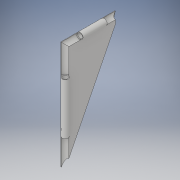
# Autodesk Inventor part: backPlate
Saved by Autodesk Inventor 2019 (Build 230136000, 136)
## iProperties
Created: 2018-07-23
Part Number: backPlate
Material: Generic
Document SubType Name: Modeling
Designer: Ge Shi
Density: 1 g/cm^3
Appearance: Default
Author: Ge Shi
Autodesk Inventor part; units mm, degrees
ref_plane "YZ Plane" through (0, 0, 0) normal (1, 0, 0) x (0, 1, 0)
ref_plane "XZ Plane" through (0, 0, 0) normal (0, 1, 0) x (-1, 0, 0)
ref_plane "XY Plane" through (0, 0, 0) normal (0, 0, 1) x (1, 0, 0)
sketch "Sketch1" plane through (0, 0, 0) normal (1, 0, 0) x (0, 1, 0)
  line L0 (-50, -25) -> (50, -25)
  line L1 (50, -25) -> (50, 25)
  line L2 (50, 25) -> (-50, 25)
  line L3 (-50, 25) -> (-50, -25)
  line L4 (-50, -25) -> (50, 25) construction
  line L5 (50, -25) -> (-50, 25) construction
  point P0 (0, 0)
  dimension "d0" = 50
  dimension "d1" = 100
  constraints: 12 end point, 2 midpoint, 2 parallel, 1 horizontal, 1 perpendicular
  measures "d0" distance of L0.end L1.end
  measures "d1" distance of L1.end L2.end
extrude "Extrusion1" add sketch "Sketch1" along normal blind 4
ref_plane "Work Plane1" through (0, 0, 25) normal (0, 1, 0) x (1, 0, 0)
ref_plane "Work Plane2" through (0, -50, 0) normal (0, 0, 1) x (1, 0, 0)
sketch "Sketch3" plane through (0, -50, 0) normal (0, 0, 1) x (1, 0, 0)
  circle A0 centre (4, 100) radius 2.25
  circle A1 centre (4, 0) radius 2.25
  circle A2 centre (4, 0) radius 2.75
  circle A3 centre (4, 100) radius 2.75
  line L0 (4, 0) -> (4, 100) projected
  circle A4 centre (4, 0) radius 3.5
  circle A5 centre (4, 100) radius 3.5
  point P0 (0, 50)
  dimension "d12" = 4.5
  dimension "d13" = 4.5
  dimension "d14" = 5.5
  dimension "d15" = 5.5
  dimension "d24" = 7
  dimension "d25" = 7
  constraints: 6 centre point, 4 coincident
  measures "d12" diameter of A0
  measures "d13" diameter of A1
  measures "d14" diameter of A2
  measures "d15" diameter of A3
  measures "d24" diameter of A4
  measures "d25" diameter of A5
sketch "Sketch2" plane through (0, 0, 25) normal (0, 1, 0) x (1, 0, 0)
  line L0 (4, 50) -> (4, 0) projected
  circle A0 centre (4, 0) radius 2.25
  circle A1 centre (4, 50) radius 2.25
  circle A2 centre (4, 0) radius 2.75
  circle A3 centre (4, 50) radius 2.75
  circle A4 centre (4, 0) radius 3.5
  circle A5 centre (4, 50) radius 3.5
  point P0 (0, 25)
  dimension "d4" = 4.5
  dimension "d5" = 4.5
  dimension "d6" = 5.5
  dimension "d7" = 5.5
  dimension "d20" = 7
  dimension "d21" = 7
  constraints: 6 centre point, 5 coincident
  measures "d4" diameter of A0
  measures "d5" diameter of A1
  measures "d6" diameter of A2
  measures "d7" diameter of A3
  measures "d20" diameter of A4
  measures "d21" diameter of A5
ref_plane "Work Plane4" through (0, -50, 25) normal (0, 0.4472136, 0.8944272) x (1, 0, 0)
extrude "Extrusion6" cut sketch "Sketch2" along normal mid plane 100 contours A0 | A1 | A2 | A3
extrude "Extrusion2" add sketch "Sketch2" along normal mid plane 47.25 contours A2 | A3
extrude "Extrusion7" cut sketch "Sketch3" along normal mid plane 50 contours A0 | A1 | A2 | A3
extrude "Extrusion4" add sketch "Sketch3" along normal mid plane 22.25 contours A2 | A3
extrude "Extrusion8" cut sketch "Sketch2" along normal blind 50 from surface at 23.625 contours A4
extrude "Extrusion9" cut sketch "Sketch2" against normal blind 50 from surface at -23.625 contours A4
extrude "Extrusion10" cut sketch "Sketch2" along normal blind 50 from surface at 23.625 contours A5
extrude "Extrusion11" cut sketch "Sketch2" against normal blind 50 from surface at -23.625 contours A5
extrude "Extrusion12" cut sketch "Sketch3" against normal blind 25 from surface at -11.125 contours A4
extrude "Extrusion13" cut sketch "Sketch3" along normal blind 25 from surface at 11.125 contours A4
extrude "Extrusion14" cut sketch "Sketch3" along normal blind 25 from surface at 11.125 contours A5
extrude "Extrusion15" cut sketch "Sketch3" against normal blind 25 from surface at -11.125 contours A5
sketch "Sketch6" plane through (0, -50, 25) normal (0, 0.4472136, 0.8944272) x (1, 0, 0)
  line L0 (4, 4.6957) -> (0, 3.4369)
  line L1 (0, 3.4369) -> (0, 108.3665)
  line L2 (0, 108.3665) -> (4, 107.1077)
  line L3 (4, 107.1077) -> (4, 4.6957)
  line L4 (4, 44.7214) -> (4, 86.983) projected
  line L5 (9.5, 0.6607) -> (-5.5, -4.0599)
  line L6 (-5.5, -4.0599) -> (-5.5, 115.8633)
  line L7 (-5.5, 115.8633) -> (9.5, 111.1427)
  line L8 (9.5, 111.1427) -> (9.5, 0.6607)
  line L9 (2, 107.7371) -> (2, 4.0663) construction
  circle A0 centre (2, 55.9017) radius 1
  line L10 (2, 79.7862) -> (2, -23.8845) construction
  circle A1 centre (2, 27.9508) radius 1
  line L11 (2, 135.6879) -> (2, 32.0172) construction
  circle A2 centre (2, 83.8525) radius 1
  line L12 (2, 107.7371) -> (2, 4.0663) construction
  circle A3 centre (2, 55.9017) radius 1
  point P0 (0, 55.9017)
  dimension "d44" = 5.5
  dimension "d47" = 2
  dimension "d50" = 27.9508
  dimension "d53" = 27.9508
  constraints: 24 end point, 4 centre point, 3 collinear, 3 midpoint, 2 vertical, 16 other
  measures "d44" distance between parallel lines of L3 L8
  measures "d47" diameter of A0
  measures "d50" distance of L9.start L10.start
  measures "d53" distance of L9.start L11.start
extrude "Extrusion16" cut sketch "Sketch6" against normal through all contours L0 L1 L2 L3 | L5 L6 L7 L8 | A0 | A1 | A2
extrude "Extrusion17" cut sketch "Sketch6" along normal blind 27.9508 contours A0 | A1 | A2
equation "\"d0\" = length"
equation "\"d1\" = height"
equation "\"d2\" = thick"
equation "\"d12\" = hingeShaft + clearance"
equation "\"d13\" = hingeShaft + clearance"
equation "\"d14\" = hingeShaftHolder"
equation "\"d15\" = hingeShaftHolder"
equation "\"d24\" = hingeShaftHolder + clearance"
equation "\"d25\" = hingeShaftHolder + clearance"
equation "\"d4\" = hingeShaft + clearance"
equation "\"d5\" = hingeShaft + clearance"
equation "\"d6\" = hingeShaftHolder"
equation "\"d7\" = hingeShaftHolder"
equation "\"d20\" = hingeShaftHolder + clearance"
equation "\"d21\" = hingeShaftHolder + clearance"
equation "\"d22\" = height"
equation "\"d26\" = length"
equation "\"d28\" = 0.5 * height"
equation "\"d30\" = 0.5 * height"
equation "\"d32\" = 0.5 * height"
equation "\"d34\" = 0.5 * height"
equation "\"d36\" = 0.5 * length"
equation "\"d38\" = 0.5 * length"
equation "\"d40\" = 0.5 * length"
equation "\"d42\" = 0.5 * length"
equation "\"d44\" = hingeShaftHolder"
equation "\"d47\" = 0.5 * thick"
equation "\"length\" = 50"
equation "\"height\" = 100"
equation "\"thick\" = 4"
equation "\"hingeShaft\" = 3"
equation "\"clearance\" = 1.5"
equation "\"hingeShaftHolder\" = 5.5"
body "Solid1"
